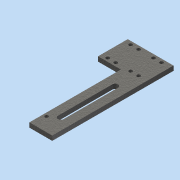
# Autodesk Inventor part: Montageplatte
Saved by Autodesk Inventor 2015 (Build 190159000, 159)
## iProperties
Created: 2017-11-12
Part Number: Montageplatte
Material: Generisch
Document SubType Name: Modeling
Designer: Christoph Soppa
Density: 1 g/cm^3
Appearance: Stahl - Guss
Author: Christoph Soppa
Autodesk Inventor part; units mm, degrees
ref_plane "YZ Plane" through (0, 0, 0) normal (1, 0, 0) x (0, 1, 0)
ref_plane "XZ Plane" through (0, 0, 0) normal (0, 1, 0) x (-1, 0, 0)
ref_plane "XY Plane" through (0, 0, 0) normal (0, 0, 1) x (1, 0, 0)
sketch "Skizze1" plane through (0, 0, 0) normal (0, 0, 1) x (1, 0, 0)
  line L0 (0, 0) -> (0, 80)
  line L1 (0, 80) -> (-20, 80)
  line L2 (-20, 80) -> (-20, 106)
  line L3 (-20, 106) -> (20, 106)
  line L4 (20, 106) -> (20, 0)
  line L5 (20, 0) -> (0, 0)
  arc A0 (7.5, 17.5) -> (12.5, 17.5) centre (10, 17.5) ccw
  arc A1 (12.5, 65) -> (7.5, 65) centre (10, 65) ccw
  line L6 (7.5, 65) -> (7.5, 17.5)
  line L7 (12.5, 65) -> (12.5, 17.5)
  dimension "d0" = 26
  dimension "d1" = 80
  dimension "d2" = 40
  dimension "d3" = 20
  dimension "d5" = 5
  dimension "d6" = 15
  dimension "d7" = 10
  dimension "d8" = 10
  dimension "d9" = 65
  dimension "d12" = 2.5
  constraints: 16 end point, 5 perpendicular, 4 point on circle, 4 tangent, 2 centre point, 1 vertical
  measures "d0" distance of L1.end L2.end
  measures "d1" distance of L0.start L0.end
  measures "d2" distance of L2.end L3.end
  measures "d3" distance of L4.end L0.start
  measures "d5" diameter of A0
  measures "d6" distance edge to line of A0 L5
  measures "d7" distance from line of L4 A1.centre
  measures "d8" distance from line of L4 A0.centre
  measures "d9" distance from line of A1.centre L5
  measures "d12" radius of A1
extrude "Extrusion1" add sketch "Skizze1" along normal blind 4
hole "Bohrung1" at (-14.5, 83, 4) direction (0, 0, -1) diameter 3 depth 8 tip angle 118
hole "Bohrung2" at (-7.5, 83, 4) direction (0, 0, -1) diameter 3 depth 8 tip angle 118
hole "Bohrung3" at (5.5, 83, 4) direction (0, 0, -1) diameter 3 depth 8 tip angle 118
hole "Bohrung4" at (12.5, 83, 4) direction (0, 0, -1) diameter 3 depth 8 tip angle 118
hole "Bohrung5" at (-14.5, 103, 4) direction (0, 0, -1) diameter 3 depth 8 tip angle 118
hole "Bohrung6" at (-7.5, 103, 4) direction (0, 0, -1) diameter 3 depth 8 tip angle 118
hole "Bohrung7" at (5.5, 103, 4) direction (0, 0, -1) diameter 3 depth 8 tip angle 118
hole "Bohrung8" at (12.5, 103, 4) direction (0, 0, -1) diameter 3 depth 8 tip angle 118
hole "Bohrung9" at (3, 12, 4) direction (0, 0, -1) diameter 3 depth 8 tip angle 118
